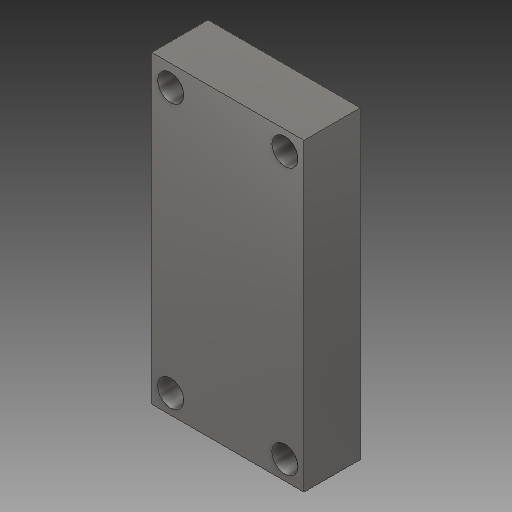
# Autodesk Inventor part: Cover Plate
Saved by Autodesk Inventor 2018 (Build 220112000, 112)
## iProperties
Created: 2017-12-21
Part Number: Cover Plate
Material: Stainless Steel
Document SubType Name: Modeling
Designer: 232963
Density: 8 g/cm^3
Appearance: Semi-Polished
Author: 232963
Autodesk Inventor part; units mm, degrees
ref_plane "YZ Plane" through (0, 0, 0) normal (1, 0, 0) x (0, 1, 0)
ref_plane "XZ Plane" through (0, 0, 0) normal (0, 1, 0) x (-1, 0, 0)
ref_plane "XY Plane" through (0, 0, 0) normal (0, 0, 1) x (1, 0, 0)
sketch "Sketch1" plane through (0, 0, 0) normal (0, 0, 1) x (1, 0, 0)
  line L0 (-12.7792, 0) -> (12.6208, 0)
  line L1 (12.6208, 0) -> (12.6208, 50.8)
  line L2 (12.6208, 50.8) -> (-12.7792, 50.8)
  line L3 (-12.7792, 50.8) -> (-12.7792, 0)
  circle A0 centre (-9.6042, 47.3128) radius 2.1844
  circle A1 centre (9.4458, 47.625) radius 2.1844
  circle A2 centre (-9.6042, 3.175) radius 2.1844
  circle A3 centre (9.4458, 3.175) radius 2.1844
  point P0 (0, 0)
  dimension "d0" = 25.4
  dimension "d1" = 50.8
  dimension "d2" = 4.3688
  dimension "d3" = 4.3688
  dimension "d4" = 4.3688
  dimension "d5" = 4.3688
  dimension "d6" = 3.175
  dimension "d7" = 3.175
  dimension "d8" = 3.175
  dimension "d9" = 3.175
  constraints: 8 end point, 4 centre point, 2 parallel, 2 vertical alignment, 1 horizontal, 1 horizontal alignment, 1 perpendicular
  measures "d0" distance of L2.end L1.end
  measures "d1" distance of L1.end L0.end
  measures "d2" diameter of A0
  measures "d3" diameter of A1
  measures "d4" diameter of A2
  measures "d5" diameter of A3
  measures "d6" distance from line of L3 A0.centre
  measures "d7" distance from line of L1 A1.centre
  measures "d8" distance from line of L2 A1.centre
  measures "d9" distance from line of L0 A3.centre
extrude "Extrusion1" add sketch "Sketch1" along normal blind 9.398
equation "\"d3\" = d2"
equation "\"d4\" = d2"
equation "\"d5\" = d2"
body "Solid1"
